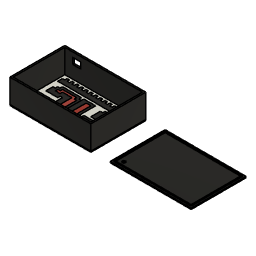
TJC-Lamp - Final (Autodesk Fusion 360 design; units mm, degrees)
Autodesk Fusion 360 part; units mm, degrees
sketch "Skizze1" plane through (0, 0, 0) normal (0, 0, 1) x (1, 0, 0)
  line L0 (-50, 50) -> (-45, 50)
  line L1 (-50, 50) -> (-50, 40)
  line L2 (-45, 50) -> (-45, 55)
  line L3 (-45, 55) -> (-40, 55)
  line L4 (-40, 55) -> (-40, 50)
  line L5 (-40, 50) -> (-35, 50)
  line L6 (-35, 50) -> (-35, 55)
  line L7 (-35, 55) -> (-30, 55)
  line L8 (-30, 55) -> (-30, 50)
  line L9 (-30, 50) -> (-25, 50)
  line L10 (-25, 50) -> (-25, 55)
  line L11 (-25, 55) -> (-20, 55)
  line L12 (-20, 55) -> (-20, 50)
  line L13 (-20, 50) -> (-15, 50)
  line L14 (-15, 50) -> (-15, 55)
  line L15 (-15, 55) -> (-10, 55)
  line L16 (-10, 55) -> (-10, 50)
  line L17 (-10, 50) -> (-5, 50)
  line L18 (-5, 50) -> (-5, 55)
  line L19 (-5, 55) -> (0, 55)
  line L20 (0, 55) -> (0, 50)
  line L21 (0, 50) -> (5, 50)
  line L22 (5, 50) -> (5, 55)
  line L23 (5, 55) -> (10, 55)
  line L24 (10, 55) -> (10, 50)
  line L25 (10, 50) -> (15, 50)
  line L26 (15, 50) -> (15, 55)
  line L27 (15, 55) -> (20, 55)
  line L28 (20, 55) -> (20, 50)
  line L29 (20, 50) -> (25, 50)
  line L30 (25, 50) -> (25, 55)
  line L31 (25, 55) -> (30, 55)
  line L32 (30, 55) -> (30, 50)
  line L33 (30, 50) -> (35, 50)
  line L34 (35, 50) -> (35, 55)
  line L35 (35, 55) -> (40, 55)
  line L36 (40, 55) -> (40, 50)
  line L37 (40, 50) -> (45, 50)
  line L38 (45, 50) -> (45, 55)
  line L39 (45, 55) -> (50, 55)
  line L40 (50, 55) -> (50, 50)
  line L41 (50, 50) -> (55, 50)
  line L42 (55, 50) -> (55, 55)
  line L43 (55, 55) -> (60, 55)
  line L44 (60, 55) -> (60, 50)
  line L45 (60, 50) -> (65, 50)
  line L46 (65, 50) -> (65, 55)
  line L47 (65, 55) -> (70, 55)
  line L48 (70, 55) -> (70, 50)
  line L49 (70, 50) -> (75, 50)
  line L50 (75, 50) -> (75, 55)
  line L51 (75, 55) -> (80, 55)
  line L52 (80, 55) -> (80, 50)
  line L53 (80, 50) -> (85, 50)
  line L54 (85, 50) -> (85, 55)
  line L55 (85, 55) -> (90, 55)
  line L56 (90, 55) -> (90, 50)
  line L57 (90, 50) -> (95, 50)
  line L58 (95, 50) -> (95, 55)
  line L59 (95, 55) -> (100, 55)
  line L60 (100, 55) -> (100, 50)
  line L61 (100, 50) -> (105, 50)
  line L62 (105, 50) -> (105, 40)
  line L63 (105, 40) -> (-50, 40)
  line L64 (-50, 40) -> (-50, 35) construction
  line L65 (-50, 35) -> (-50, 15)
  line L66 (-50, 15) -> (-35, 15)
  line L67 (-50, 35) -> (0, 35)
  line L68 (-35, 15) -> (-35, -20)
  line L69 (-35, -20) -> (-30, -20)
  line L70 (-30, -20) -> (-30, -25)
  line L71 (-30, -25) -> (-10, -25)
  line L72 (-10, -25) -> (-10, 10)
  line L73 (-10, 10) -> (5, 10)
  line L74 (5, 10) -> (5, 30)
  line L75 (5, 30) -> (0, 30)
  line L76 (0, 30) -> (0, 35)
  line L77 (-5, 30) -> (-45, 30)
  line L78 (-45, 30) -> (-45, 20)
  line L79 (-5, 30) -> (-5, 20)
  line L80 (-5, 20) -> (-20, 20)
  line L81 (-45, 20) -> (-30, 20)
  line L82 (-30, 20) -> (-30, -15)
  line L83 (-30, -15) -> (-20, -15)
  line L84 (-20, -15) -> (-20, 20)
  line L85 (-10, -15) -> (-5, -15)
  line L86 (-5, -15) -> (-5, -20)
  line L87 (-5, -20) -> (0, -20)
  line L88 (0, -20) -> (0, -25)
  line L89 (-10, -15) -> (-10, 5)
  line L90 (-10, 5) -> (15, 5)
  line L91 (15, 5) -> (15, 0)
  line L92 (15, 0) -> (20, 0)
  line L93 (20, 0) -> (20, 35)
  line L94 (20, 35) -> (45, 35)
  line L95 (45, 35) -> (45, -15)
  line L96 (45, -15) -> (45, -20)
  line L97 (45, -20) -> (40, -20)
  line L98 (40, -20) -> (40, -25)
  line L99 (40, -25) -> (0, -25)
  line L100 (-5, -10) -> (-5, 0)
  line L101 (-5, 0) -> (5, 0)
  line L102 (5, 0) -> (5, -10)
  line L103 (-5, -10) -> (0, -10)
  line L104 (0, -10) -> (0, -15)
  line L105 (0, -15) -> (5, -15)
  line L106 (5, -15) -> (25, -15)
  line L107 (5, -10) -> (25, -10)
  line L108 (25, -10) -> (25, 30)
  line L109 (25, 30) -> (35, 30)
  line L110 (35, 30) -> (35, -10)
  line L111 (35, -10) -> (30, -10)
  line L112 (30, -10) -> (30, -15)
  line L113 (30, -15) -> (25, -15)
  line L114 (50, -15) -> (45, -15)
  line L115 (45, -15) -> (45, 30)
  line L116 (45, 30) -> (50, 30)
  line L117 (50, 30) -> (50, 35)
  line L118 (50, 35) -> (90, 35)
  line L119 (90, 35) -> (90, 30)
  line L120 (90, 30) -> (95, 30)
  line L121 (95, 30) -> (95, 25)
  line L122 (95, 25) -> (100, 25)
  line L123 (100, 25) -> (100, 10)
  line L124 (50, -15) -> (50, -20)
  line L125 (50, -20) -> (55, -20)
  line L126 (55, -20) -> (55, -25)
  line L127 (55, -25) -> (95, -25)
  line L128 (95, -25) -> (95, -20)
  line L129 (95, -20) -> (100, -20)
  line L130 (100, -20) -> (100, -5)
  line L131 (100, -5) -> (95, -5)
  line L132 (95, -5) -> (95, 0)
  line L133 (95, 0) -> (75, 0)
  line L134 (75, 0) -> (75, -5)
  line L135 (75, -5) -> (70, -5)
  line L136 (70, -5) -> (70, 15)
  line L137 (70, 15) -> (75, 15)
  line L138 (75, 15) -> (75, 10)
  line L139 (75, 10) -> (100, 10)
  line L140 (55, 30) -> (55, 25)
  line L141 (55, 25) -> (50, 25)
  line L142 (50, 25) -> (50, -10)
  line L143 (55, 30) -> (85, 30)
  line L144 (85, 30) -> (85, 25)
  line L145 (85, 25) -> (90, 25)
  line L146 (90, 25) -> (90, 20)
  line L147 (90, 20) -> (80, 20)
  line L148 (80, 20) -> (80, 25)
  line L149 (80, 25) -> (60, 25)
  line L150 (60, 25) -> (60, -10)
  line L151 (50, -10) -> (55, -10)
  line L152 (55, -10) -> (55, -15)
  line L153 (60, -10) -> (80, -10)
  line L154 (80, -10) -> (80, -5)
  line L155 (80, -5) -> (90, -5)
  line L156 (90, -5) -> (90, -10)
  line L157 (90, -10) -> (85, -10)
  line L158 (85, -10) -> (85, -15)
  line L159 (85, -15) -> (55, -15)
  line L160 (-50, 40) -> (-50, -30) construction
  line L161 (105, -30) -> (105, 40) construction
  line L162 (-50, -30) -> (105, -30)
  line L163 (105, -30) -> (105, -40)
  line L164 (-50, -30) -> (-50, -40)
  line L165 (-50, -40) -> (-45, -40)
  line L166 (-45, -40) -> (-45, -45)
  line L167 (-45, -45) -> (-40, -45)
  line L168 (-40, -45) -> (-40, -40)
  line L169 (-40, -40) -> (-35, -40)
  line L170 (-35, -40) -> (-35, -45)
  line L171 (-35, -45) -> (-30, -45)
  line L172 (-30, -45) -> (-30, -40)
  line L173 (-30, -40) -> (-25, -40)
  line L174 (-25, -40) -> (-25, -45)
  line L175 (-25, -45) -> (-20, -45)
  line L176 (-20, -45) -> (-20, -40)
  line L177 (-20, -40) -> (-15, -40)
  line L178 (-15, -40) -> (-15, -45)
  line L179 (-15, -45) -> (-10, -45)
  line L180 (-10, -45) -> (-10, -40)
  line L181 (-10, -40) -> (-5, -40)
  line L182 (-5, -40) -> (-5, -45)
  line L183 (-5, -45) -> (0, -45)
  line L184 (0, -45) -> (0, -40)
  line L185 (0, -40) -> (5, -40)
  line L186 (5, -40) -> (5, -45)
  line L187 (5, -45) -> (10, -45)
  line L188 (10, -45) -> (10, -40)
  line L189 (10, -40) -> (15, -40)
  line L190 (15, -40) -> (15, -45)
  line L191 (15, -45) -> (20, -45)
  line L192 (20, -45) -> (20, -40)
  line L193 (20, -40) -> (25, -40)
  line L194 (25, -40) -> (25, -45)
  line L195 (25, -45) -> (30, -45)
  line L196 (30, -45) -> (30, -40)
  line L197 (30, -40) -> (35, -40)
  line L198 (35, -40) -> (35, -45)
  line L199 (35, -45) -> (40, -45)
  line L200 (40, -45) -> (40, -40)
  line L201 (40, -40) -> (45, -40)
  line L202 (45, -40) -> (45, -45)
  line L203 (45, -45) -> (50, -45)
  line L204 (50, -45) -> (50, -40)
  line L205 (50, -40) -> (55, -40)
  line L206 (55, -40) -> (55, -45)
  line L207 (55, -45) -> (60, -45)
  line L208 (60, -45) -> (60, -40)
  line L209 (60, -40) -> (65, -40)
  line L210 (65, -40) -> (65, -45)
  line L211 (65, -45) -> (70, -45)
  line L212 (70, -45) -> (70, -40)
  line L213 (70, -40) -> (75, -40)
  line L214 (75, -40) -> (75, -45)
  line L215 (75, -45) -> (80, -45)
  line L216 (80, -45) -> (80, -40)
  line L217 (80, -40) -> (85, -40)
  line L218 (85, -40) -> (85, -45)
  line L219 (85, -45) -> (90, -45)
  line L220 (90, -45) -> (90, -40)
  line L221 (90, -40) -> (95, -40)
  line L222 (95, -40) -> (95, -45)
  line L223 (95, -45) -> (100, -45)
  line L224 (100, -45) -> (100, -40)
  line L225 (100, -40) -> (105, -40)
  line L226 (-58, -53) -> (113, -53)
  line L227 (113, -53) -> (113, 63)
  line L228 (113, 63) -> (-58, 63)
  line L229 (-58, 63) -> (-58, -53)
  line L230 (360.6079, -53.7014) -> (360.6079, 62.2986)
  line L231 (360.6079, 62.2986) -> (189.6079, 62.2986)
  line L232 (189.6079, 62.2986) -> (189.6079, -53.7014)
  line L233 (189.6079, -53.7014) -> (360.6079, -53.7014)
  line L234 (357.1079, -50.2014) -> (357.1079, 58.7986)
  line L235 (357.1079, 58.7986) -> (193.1079, 58.7986)
  line L236 (193.1079, 58.7986) -> (193.1079, -50.2014)
  line L237 (193.1079, -50.2014) -> (357.1079, -50.2014)
  line L238 (195.1079, -48.2014) -> (355.1079, -48.2014)
  line L239 (355.1079, -48.2014) -> (355.1079, 56.7986)
  line L240 (355.1079, 56.7986) -> (195.1079, 56.7986)
  line L241 (195.1079, 56.7986) -> (195.1079, -48.2014)
  circle A0 centre (205, -40) radius 3.5
  line L242 (-54.5, -49.5) -> (109.5, -49.5)
  line L243 (109.5, -49.5) -> (109.5, 59.5)
  line L244 (109.5, 59.5) -> (-54.5, 59.5)
  line L245 (-54.5, 59.5) -> (-54.5, -49.5)
  line L246 (107.5, -47.5) -> (107.5, 57.5)
  line L247 (107.5, 57.5) -> (-52.5, 57.5)
  line L248 (-52.5, 57.5) -> (-52.5, -47.5)
  line L249 (-52.5, -47.5) -> (107.5, -47.5)
  dimension "d1" = 5
  dimension "d2" = 10
  dimension "d3" = 15
  dimension "d4" = 50
  dimension "d5" = 35
  dimension "d6" = 20
  dimension "d7" = 35
  dimension "d8" = 15
  dimension "d9" = 20
  dimension "d10" = 35
  dimension "d11" = 25
  dimension "d12" = 35
  dimension "d13" = 25
  dimension "d14" = 50
  dimension "d18" = 20
  dimension "d19" = 40
  dimension "d20" = 10
  dimension "d21" = 40
  dimension "d22" = 40
  dimension "d23" = 40
  dimension "d24" = 20
  dimension "d25" = 20
  dimension "d26" = 30
  dimension "d29" = -3.5
  dimension "d30" = -5.5
  dimension "d31" = 7
  dimension "d38" = -3.5
  dimension "d39" = -5.5
  constraint horizontal L0
  constraint perpendicular L0 L1
  constraint perpendicular L0 L2
  constraint perpendicular L2 L3
  constraint perpendicular L3 L4
  constraint perpendicular L4 L5
  constraint perpendicular L3 L6
  constraint perpendicular L4 L7
  constraint perpendicular L7 L8
  constraint perpendicular L8 L9
  constraint perpendicular L9 L10
  constraint perpendicular L10 L11
  constraint perpendicular L11 L12
  constraint perpendicular L12 L13
  constraint perpendicular L11 L14
  constraint perpendicular L12 L15
  constraint perpendicular L11 L16
  constraint perpendicular L12 L17
  constraint perpendicular L11 L18
  constraint perpendicular L18 L19
  constraint perpendicular L19 L20
  constraint perpendicular L20 L21
  constraint perpendicular L21 L22
  constraint perpendicular L22 L23
  constraint perpendicular L23 L24
  constraint perpendicular L22 L25
  constraint perpendicular L25 L26
  constraint perpendicular L26 L27
  constraint perpendicular L27 L28
  constraint perpendicular L28 L29
  constraint perpendicular L27 L30
  constraint perpendicular L30 L31
  constraint perpendicular L31 L32
  constraint perpendicular L32 L33
  constraint perpendicular L33 L34
  constraint perpendicular L34 L35
  constraint perpendicular L35 L36
  constraint perpendicular L36 L37
  constraint perpendicular L35 L38
  constraint perpendicular L38 L39
  constraint perpendicular L39 L40
  constraint perpendicular L40 L41
  constraint perpendicular L41 L42
  constraint perpendicular L42 L43
  constraint perpendicular L43 L44
  constraint perpendicular L44 L45
  constraint perpendicular L43 L46
  constraint perpendicular L46 L47
  constraint perpendicular L47 L48
  constraint perpendicular L46 L49
  constraint perpendicular L49 L50
  constraint perpendicular L50 L51
  constraint perpendicular L51 L52
  constraint perpendicular L52 L53
  constraint perpendicular L51 L54
  constraint perpendicular L54 L55
  constraint perpendicular L55 L56
  constraint perpendicular L56 L57
  constraint perpendicular L57 L58
  constraint perpendicular L58 L59
  constraint perpendicular L59 L60
  constraint perpendicular L58 L61
  constraint perpendicular L59 L62
  constraint perpendicular L63 L64
  constraint perpendicular L65 L66
  constraint perpendicular L65 L67
  constraint perpendicular L66 L68
  constraint perpendicular L68 L69
  constraint perpendicular L69 L70
  constraint perpendicular L70 L71
  constraint perpendicular L71 L72
  constraint perpendicular L72 L73
  constraint perpendicular L73 L74
  constraint perpendicular L74 L75
  constraint perpendicular L65 L77
  constraint perpendicular L66 L78
  constraint perpendicular L77 L79
  constraint perpendicular L79 L80
  constraint perpendicular L78 L81
  constraint perpendicular L81 L82
  constraint perpendicular L82 L83
  constraint perpendicular L80 L84
  constraint horizontal L85
  constraint perpendicular L85 L86
  constraint perpendicular L86 L87
  constraint perpendicular L87 L88
  constraint coincident L72 L89.end
  constraint perpendicular L72 L90
  constraint perpendicular L90 L91
  constraint perpendicular L91 L92
  constraint perpendicular L92 L93
  constraint horizontal L94
  constraint perpendicular L93 L94
  constraint perpendicular L94 L95
  constraint parallel L95 L96
  constraint perpendicular L96 L97
  constraint perpendicular L97 L98
  constraint perpendicular L88 L99
  constraint perpendicular L73 L100
  constraint perpendicular L100 L101
  constraint perpendicular L101 L102
  constraint perpendicular L100 L103
  constraint perpendicular L103 L104
  constraint perpendicular L104 L105
  constraint parallel L105 L106
  constraint perpendicular L102 L107
  constraint perpendicular L107 L108
  constraint perpendicular L108 L109
  constraint perpendicular L109 L110
  constraint perpendicular L110 L111
  constraint perpendicular L111 L112
  constraint perpendicular L112 L113
  constraint coincident L95 L115.end
  constraint perpendicular L115 L116
  constraint perpendicular L116 L117
  constraint perpendicular L117 L118
  constraint perpendicular L118 L119
  constraint perpendicular L119 L120
  constraint perpendicular L120 L121
  constraint perpendicular L119 L122
  constraint perpendicular L122 L123
  constraint perpendicular L114 L124
  constraint perpendicular L124 L125
  constraint perpendicular L114 L126
  constraint perpendicular L126 L127
  constraint perpendicular L127 L128
  constraint perpendicular L128 L129
  constraint perpendicular L129 L130
  constraint perpendicular L130 L131
  constraint perpendicular L131 L132
  constraint perpendicular L132 L133
  constraint perpendicular L133 L134
  constraint perpendicular L134 L135
  constraint perpendicular L135 L136
  constraint perpendicular L136 L137
  constraint perpendicular L137 L138
  constraint perpendicular L123 L139
  constraint perpendicular L116 L140
  constraint perpendicular L140 L141
  constraint perpendicular L141 L142
  constraint perpendicular L140 L143
  constraint perpendicular L143 L144
  constraint perpendicular L144 L145
  constraint perpendicular L145 L146
  constraint perpendicular L146 L147
  constraint perpendicular L147 L148
  constraint perpendicular L146 L149
  constraint perpendicular L149 L150
  constraint perpendicular L142 L151
  constraint perpendicular L151 L152
  constraint perpendicular L150 L153
  constraint perpendicular L153 L154
  constraint perpendicular L150 L155
  constraint perpendicular L155 L156
  constraint perpendicular L156 L157
  constraint perpendicular L157 L158
  constraint perpendicular L152 L159
  constraint parallel L62 L161
  constraint perpendicular L161 L162
  constraint perpendicular L162 L163
  constraint perpendicular L162 L164
  constraint perpendicular L164 L165
  constraint perpendicular L165 L166
  constraint perpendicular L166 L167
  constraint perpendicular L167 L168
  constraint perpendicular L168 L169
  constraint perpendicular L169 L170
  constraint perpendicular L170 L171
  constraint perpendicular L171 L172
  constraint perpendicular L172 L173
  constraint perpendicular L173 L174
  constraint perpendicular L172 L175
  constraint perpendicular L175 L176
  constraint perpendicular L176 L177
  constraint perpendicular L177 L178
  constraint perpendicular L178 L179
  constraint perpendicular L179 L180
  constraint perpendicular L180 L181
  constraint perpendicular L181 L182
  constraint perpendicular L180 L183
  constraint perpendicular L183 L184
  constraint perpendicular L184 L185
  constraint perpendicular L183 L186
  constraint perpendicular L186 L187
  constraint perpendicular L187 L188
  constraint perpendicular L188 L189
  constraint perpendicular L189 L190
  constraint perpendicular L190 L191
  constraint perpendicular L191 L192
  constraint perpendicular L192 L193
  constraint perpendicular L191 L194
  constraint perpendicular L194 L195
  constraint perpendicular L195 L196
  constraint perpendicular L196 L197
  constraint perpendicular L195 L198
  constraint perpendicular L196 L199
  constraint perpendicular L195 L200
  constraint perpendicular L200 L201
  constraint perpendicular L201 L202
  constraint perpendicular L202 L203
  constraint perpendicular L203 L204
  constraint perpendicular L204 L205
  constraint perpendicular L203 L206
  constraint perpendicular L206 L207
  constraint perpendicular L203 L208
  constraint perpendicular L208 L209
  constraint perpendicular L209 L210
  constraint perpendicular L210 L211
  constraint perpendicular L211 L212
  constraint perpendicular L212 L213
  constraint perpendicular L213 L214
  constraint perpendicular L212 L215
  constraint perpendicular L213 L216
  constraint perpendicular L216 L217
  constraint perpendicular L213 L218
  constraint perpendicular L218 L219
  constraint perpendicular L219 L220
  constraint perpendicular L220 L221
  constraint perpendicular L219 L222
  constraint perpendicular L222 L223
  constraint perpendicular L223 L224
  measures "d1" distance of L0.start L0.end
  measures "d2" distance of L0.start L1.end
  measures "d3" distance of L65.end L66.end
  measures "d4" distance of L64.end L67.end
  measures "d5" distance of L66.end L68.end
  measures "d6" distance of L70.end L71.end
  measures "d7" distance of L71.end L72.end
  measures "d8" distance of L72.end L73.end
  measures "d9" distance of L73.end L74.end
  measures "d10" distance of L81.end L82.end
  measures "d11" distance of L89.end L90.end
  measures "d12" distance of L92.end L93.end
  measures "d13" distance of L93.end L94.end
  measures "d14" distance of L94.end L95.end
  measures "d18" distance of L102.end L107.end
  measures "d19" distance of L107.end L108.end
  measures "d20" distance of L108.end L109.end
  measures "d21" distance of L109.end L110.end
  measures "d22" distance of L117.end L118.end
  measures "d23" distance of L126.end L127.end
  measures "d24" distance of L132.end L133.end
  measures "d25" distance of L135.end L136.end
  measures "d26" distance of L140.start L143.end
  measures "d31" diameter of A0
extrude "Extrusion1" add sketch "Skizze1" along normal blind 2.5 contours L238 L239 L240 L241 makes body 1
extrude "Extrusion2" add sketch "Skizze1" along normal blind 3.5 contours L234 L235 L236 L237 bodies 1
extrude "Extrusion3" add sketch "Skizze1" along normal blind 2.5 contours L230 L231 L232 L233 bodies 1
extrude "Extrusion4" add sketch "Skizze1" along normal blind 2 separate body contours L0 L1 L2 L3 L4 L5 L6 L7 L8 L9 L10 L11 L12 L13 L14 L15 L16 L17 L18 L19 L20 L21 L22 L23 L24 L25 L26 L27 L28 L29 L30 L31 L32 L33 L34 L35 L36 L37 L38 L39 L40 L41 L42 L43 L44 L45 L46 L47 L48 L49 L50 L51 L52 L53 L54 L55 L56 L57 L58 L59 L60 L61 L62 L63 | L65 L66 L67 L68 L69 L70 L71 L72 L73 L74 L75 L76 L89 | L72 L85 L86 L87 L88 L89 L90 L91 L92 L93 L94 L95 L96 L97 L98 L99 L115 | L140 L141 L142 L143 L144 L145 L146 L147 L148 L149 L150 L151 L152 L153 L154 L155 L156 L157 L158 L159 | L162 L163 L164 L165 L166 L167 L168 L169 L170 L171 L172 L173 L174 L175 L176 L177 L178 L179 L180 L181 L182 L183 L184 L185 L186 L187 L188 L189 L190 L191 L192 L193 L194 L195 L196 L197 L198 L199 L200 L201 L202 L203 L204 L205 L206 L207 L208 L209 L210 L211 L212 L213 L214 L215 L216 L217 L218 L219 L220 L221 L222 L223 L224 L225 makes body 2 at (26.6667, 43.3333, 0) makes body 3 at (15, -33.3333, 0) makes body 4 at (41.6667, 1.6667, 0) makes body 5 at (73.3333, -13.3333, 0)
extrude "Extrusion5" add sketch "Skizze1" along normal blind 2 separate body contours L242 L243 L244 L245 | L246 L247 L248 L249 makes body 6
extrude "Extrusion6" add sketch "Skizze1" along normal blind 2 separate body contours L95 L114 L115 L116 L117 L118 L119 L120 L121 L122 L123 L124 L125 L126 L127 L128 L129 L130 L131 L132 L133 L134 L135 L136 L137 L138 L139 | L77 L78 L79 L80 L81 L82 L83 L84 | L100 L101 L102 L103 L104 L105 L106 L107 L108 L109 L110 L111 L112 L113 makes body 7 at (78.3333, -21.6667, 0) makes body 8 at (30, 16.6667, 0) makes body 9 at (-26.6667, 26.6667, 0)
extrude "Extrusion7" add sketch "Skizze1" against normal blind 50 separate body contours L226 L227 L228 L229 makes body 10
extrude "Extrusion8" add sketch "Skizze1" along normal blind 2 separate body contours L226 L227 L228 L229 makes body 11
sketch "Skizze2" plane through (0, 63, 0) normal (0, 1, 0) x (-1, 0, 0)
  line L0 (58, 0) -> (-113, 0)
  line L1 (-113, 0) -> (-113, -50)
  line L2 (-113, -50) -> (58, -50)
  line L3 (58, -50) -> (58, 0)
  line L4 (-93, -40) -> (-76, -40)
  line L5 (-76, -40) -> (-76, -27)
  line L6 (-76, -27) -> (-93, -27)
  line L7 (-93, -27) -> (-93, -40)
  dimension "d50" = 17
  dimension "d51" = 13
  dimension "d52" = 20
  dimension "d53" = 10
  constraint horizontal L4
  constraint vertical L5
  constraint horizontal L6
  constraint vertical L7
  measures "d50" distance of L4.start L4.end
  measures "d51" distance of L4.start L6.end
  measures "d52" distance of L1 L7
  measures "d53" distance of L2 L4
extrude "Extrusion9" cut sketch "Skizze2" against normal blind 5 contours L4 L5 L6 L7 bodies 10
move_body "Verschieben1" bodies 2 8 10 6 9 11 7 5 4 3 to x (-1, 0, 0) y (0, 1, 0) z (0, 0, -1) at (-100, 0, 0)
move_body "Verschieben2" bodies 10 11 5 8 7 4 6 2 9 3 to x (1, 0, 0) y (0, 1, 0) z (0, 0, 1) at (190, 0, 0)
equation "d3 = ( 3 * 5 ) * 1 mm"
equation "d4 = ( 10 * 5 ) * 1 mm"
equation "d5 = ( 7 * 5 ) * 1 mm"
equation "d6 = ( 4 * 5 ) * 1 mm"
equation "d7 = ( 7 * 5 ) * 1 mm"
equation "d8 = ( 3 * 5 ) * 1 mm"
equation "d9 = ( 4 * 5 ) * 1 mm"
equation "d10 = ( 7 * 5 ) * 1 mm"
equation "d11 = ( 5 * 5 ) * 1 mm"
equation "d12 = ( 7 * 5 ) * 1 mm"
equation "d13 = ( 5 * 5 ) * 1 mm"
equation "d14 = ( 5 * 10 ) * 1 mm"
equation "d19 = ( 8 * 5 ) * 1 mm"
equation "d21 = ( 8 * 5 ) * 1 mm"
equation "d22 = ( 8 * 5 ) * 1 mm"
equation "d23 = ( 8 * 5 ) * 1 mm"
equation "d26 = ( 6 * 5 ) * 1 mm"
